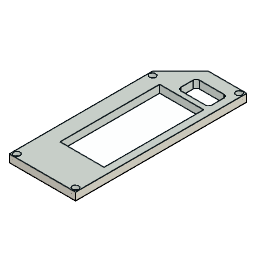
case top v17 (Autodesk Fusion 360 design; units mm, degrees)
Autodesk Fusion 360 part; units mm, degrees
box "BoxPrimitive1" add length 111 width 43 height 5 placed x (0, 1, 0) y (-1, 0, 0) z (0, 0, 1) at (43.0003, 0, 0)
sketch "Sketch6" plane through (0, 0, 0) normal (0, 0, -1) x (1, 0, 0)
  line L0 (0.0003, -111) -> (43.0003, -111)
  line L1 (43.0003, -111) -> (43.0003, 0)
  line L2 (43.0003, 0) -> (0.0003, 0)
  line L3 (0.0003, 0) -> (0.0003, -111)
  line L4 (0.0003, -93) -> (18.0003, -111)
  line L5 (6.5003, -22.25) -> (41.5003, -22.25) construction
  line L6 (41.5003, -22.25) -> (41.5003, -88.75) construction
  line L7 (41.5003, -88.75) -> (6.5003, -88.75) construction
  line L8 (6.5003, -88.75) -> (6.5003, -22.25) construction
  line L9 (6.5003, -22.25) -> (41.5003, -88.75) construction
  line L10 (6.5003, -88.75) -> (41.5003, -22.25) construction
  circle A0 centre (8.2003, -23.95) radius 0.8
  line L11 (38.2503, -87.75) -> (9.7503, -87.75)
  line L12 (9.7503, -87.75) -> (9.7503, -23.25)
  line L13 (9.7503, -23.25) -> (38.2503, -23.25)
  line L14 (38.2503, -23.25) -> (38.2503, -87.75)
  line L15 (38.2503, -87.75) -> (9.7503, -23.25) construction
  line L16 (9.7503, -87.75) -> (38.2503, -23.25) construction
  line L17 (18.2503, -91) -> (38.2503, -91)
  line L18 (38.2503, -91) -> (38.2503, -103)
  line L19 (38.2503, -103) -> (18.2503, -103)
  line L20 (18.2503, -103) -> (18.2503, -91)
  circle A1 centre (2.5003, -2.5) radius 1.2
  circle A2 centre (40.5003, -2.5) radius 1.2
  circle A3 centre (40.5003, -108.5) radius 1.2
  circle A4 centre (2.5003, -90.5) radius 1.2
  line L21 (24.0003, -111) -> (24.0003, 0) construction
  line L22 (0.0003, -55.5) -> (43.0003, -55.5) construction
  circle A5 centre (8.2003, -87.05) radius 0.8
  circle A6 centre (39.8003, -23.95) radius 0.8
  circle A7 centre (39.8003, -87.05) radius 0.8
  line L23 (18.2503, -91) -> (38.2503, -103) construction
  line L24 (38.2503, -91) -> (18.2503, -103) construction
  point P0 (24.0003, -55.5)
  point P1 (24.0003, -55.5)
  point P2 (24.0003, -55.5)
  point P3 (24.0003, -55.5)
  point P4 (28.2503, -97)
  dimension "d7" = 45
  dimension "d8" = 35
  dimension "d9" = 66.5
  dimension "d11" = 1.6
  dimension "d12" = 1.7
  dimension "d13" = 1.7
  dimension "d14" = 28.5
  dimension "d15" = 64.5
  dimension "d17" = 2.4
  dimension "d18" = 2.5
  dimension "d19" = 2.5
  dimension "d21" = 2.4
  dimension "d22" = 2.5
  dimension "d23" = 2.5
  dimension "d24" = 2.4
  dimension "d25" = 2.5
  dimension "d26" = 2.5
  dimension "d38" = 93
  dimension "d39" = 4.75
  dimension "d42" = 20
  dimension "d43" = 12
  dimension "d47" = 55.5
  dimension "d48" = 19
  dimension "d51" = 2.5
  dimension "d52" = 2.5
  dimension "d53" = 2.4
  dimension "d56" = 3.25
  constraint coincident L3 L4.start
  constraint coincident L0 L4.end
  constraint horizontal L5
  constraint vertical L6
  constraint horizontal L7
  constraint vertical L8
  constraint midpoint L10 P3
  constraint coincident P3 P2
  constraint horizontal L11
  constraint perpendicular L11 L12
  constraint parallel L11 L13
  constraint parallel L12 L14
  constraint coincident L15 P3
  constraint coincident L16 P3
  constraint horizontal L17
  constraint vertical L18
  constraint horizontal L19
  constraint vertical L20
  constraint coincident L0 L21.start
  constraint coincident L2 L21.end
  constraint perpendicular L2 L21
  constraint coincident L3 L22.start
  constraint coincident L1 L22.end
  constraint perpendicular L1 L22
  constraint coincident L21 P3
  constraint coincident L22 P3
  constraint symmetric A0 L22 A5
  constraint symmetric A0 L21 A6
  constraint symmetric L21 A5 A7
  constraint midpoint L23 P4
  measures "d7" angle of L3 L4
  measures "d8" distance of L5.start L5.end
  measures "d9" distance of L5.start L7.end
  measures "d11" diameter of A0
  measures "d12" distance of L5 A0.centre
  measures "d13" distance of L8 A0.centre
  measures "d14" distance of L11.start L11.end
  measures "d15" distance of L11.start L13.end
  measures "d17" diameter of A1
  measures "d18" distance of L3 A1.centre
  measures "d19" distance of L2 A1.centre
  measures "d21" diameter of A3
  measures "d22" distance of L1 A3.centre
  measures "d23" distance of L0 A3.centre
  measures "d24" diameter of A4
  measures "d25" distance of L3 A4.centre
  measures "d26" vertical distance of L4.start A4.centre
  measures "d38" vertical distance of origin L4.start
  measures "d39" distance of L1 L18
  measures "d42" distance of L17.start L17.end
  measures "d43" distance of L17.end L18.end
  measures "d47" distance of L2 L22
  measures "d48" distance of L1 L21
  measures "d51" distance of L2 A2.centre
  measures "d52" distance of L1 A2.centre
  measures "d53" diameter of A2
  measures "d56" distance of L11 L17
extrude "Extrude1" cut sketch "Sketch6" against normal through all contours L0 L3 L4 | L11 L12 L13 L14 | L17 L18 L19 L20 | A1 | A2 | A3 | A4
extrude "Extrude4" cut sketch "Sketch6" against normal blind 4 contours A0 | A5 | A6 | A7
thread "Thread2" "ISO Metric profile 2.0 M2x0.4 M2x0.4 6H" major diameter 2.074 minor diameter 1.623 pitch 0.4 angle 60 resizes the face on face at (39.8202, 23.1502, 2.6667) on face at (40.4829, 86.6329, 2.6667) on face at (7.4977, 86.6674, 2.6667) on face at (8.9993, 23.9101, 1.3333)
sketch "Sketch9" plane through (0, 0, 5) normal (0, 0, 1) x (-1, 0, 0)
  line L0 (-18.0003, -111) -> (-0.0003, -93)
  line L1 (-0.0003, -93) -> (-0.0003, 0)
  line L2 (-0.0003, 0) -> (-43.0003, 0)
  line L3 (-43.0003, 0) -> (-43.0003, -111)
  line L4 (-43.0003, -111) -> (-18.0003, -111)
  circle A0 centre (-40.5003, -108.5) radius 1.2
  line L5 (-18.2503, -91) -> (-18.2503, -103)
  line L6 (-18.2503, -103) -> (-38.2503, -103)
  line L7 (-38.2503, -103) -> (-38.2503, -91)
  line L8 (-38.2503, -91) -> (-18.2503, -91)
  circle A1 centre (-2.5003, -90.5) radius 1.2
  circle A2 centre (-40.5003, -2.5) radius 1.2
  line L9 (-38.2503, -87.75) -> (-38.2503, -23.25)
  line L10 (-38.2503, -23.25) -> (-9.7503, -23.25)
  line L11 (-9.7503, -23.25) -> (-9.7503, -87.75)
  line L12 (-9.7503, -87.75) -> (-38.2503, -87.75)
  circle A3 centre (-2.5003, -2.5) radius 1.2
  circle A4 centre (-2.5003, -2.5) radius 2
  circle A5 centre (-40.5003, -2.5) radius 2
  circle A6 centre (-2.5003, -90.5) radius 2
  circle A7 centre (-40.5003, -108.5) radius 2
  dimension "d32" = 4
  dimension "d33" = 4
  dimension "d34" = 4
  dimension "d35" = 4
  constraint concentric A3 A4
  constraint concentric A2 A5
  constraint concentric A1 A6
  constraint concentric A0 A7
  measures "d32" diameter of A4
  measures "d33" diameter of A5
  measures "d34" diameter of A6
  measures "d35" diameter of A7
extrude "Extrude3" cut sketch "Sketch9" against normal blind 2.5 contours A4 | A5 | A6 | A7
sketch "Sketch10" plane through (0, 0, 5) normal (0, 0, 1) x (-1, 0, 0)
  line L0 (-38.2503, -87.75) -> (-38.2503, -23.25)
  line L1 (-38.2503, -23.25) -> (-9.7503, -23.25)
  line L2 (-9.7503, -23.25) -> (-9.7503, -87.75)
  line L3 (-9.7503, -87.75) -> (-38.2503, -87.75)
  line L4 (-18.2503, -91) -> (-18.2503, -103)
  line L5 (-18.2503, -103) -> (-38.2503, -103)
  line L6 (-38.2503, -103) -> (-38.2503, -91)
  line L7 (-38.2503, -91) -> (-18.2503, -91)
  line L8 (-18.0003, -111) -> (-0.0003, -93)
  line L9 (-0.0003, -93) -> (-0.0003, 0)
  line L10 (-0.0003, 0) -> (-43.0003, 0)
  line L11 (-43.0003, 0) -> (-43.0003, -111)
  line L12 (-43.0003, -111) -> (-18.0003, -111)
  circle A0 centre (-40.5003, -108.5) radius 2
  circle A1 centre (-2.5003, -2.5) radius 2
  circle A2 centre (-2.5003, -90.5) radius 2
  circle A3 centre (-40.5003, -2.5) radius 2
fillet "Fillet1" radius 2 4 edges at (38.2503, 91, 2.5) (18.2503, 91, 2.5) (38.2503, 103, 2.5) (18.2503, 103, 2.5)
